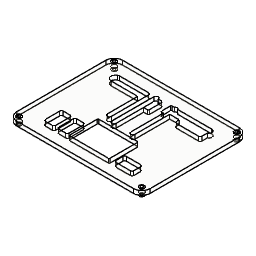
CASE TAMPA (Autodesk Fusion 360 design; units mm, degrees)
Autodesk Fusion 360 part; units mm, degrees
sketch "Esboço1" plane through (0, 0, 0) normal (0, 0, 1) x (1, 0, 0)
  arc A0 through (-111.4942, 26.079, 1.5525) (-112.9084, 25.4932, 1.5525) (-113.4942, 24.079, 1.5525)
  line L0 (-107.2442, 26.079, 1.5525) -> (-102.9942, 26.079, 1.5525)
  line L1 (-126.339, 4.5975, 1.5525) -> (-119.189, 4.5975, 1.5525)
  line L2 (-155, 19.05, 1.5525) -> (-155, -2.46, 1.5525)
  line L3 (-126.339, 4.5975, 1.5525) -> (-127.689, 4.5975, 1.5525)
  line L4 (-117.189, 6.5975, 1.5525) -> (-117.189, 6.7613, 1.5525)
  arc A1 through (-117.189, 24.079, 1.5525) (-117.7748, 25.4932, 1.5525) (-119.189, 26.079, 1.5525)
  arc A2 through (-127.689, 26.079, 1.5525) (-129.1032, 25.4932, 1.5525) (-129.689, 24.079, 1.5525)
  arc A3 through (-119.189, 4.5975, 1.5525) (-117.7748, 5.1833, 1.5525) (-117.189, 6.5975, 1.5525)
  line L5 (-129.689, 24.079, 1.5525) -> (-129.689, 6.5975, 1.5525)
  arc A4 through (-129.689, 6.5975, 1.5525) (-129.1032, 5.1833, 1.5525) (-127.689, 4.5975, 1.5525)
  arc A5 through (-44.2048, 6.3065, 1.5525) (-43.619, 4.8923, 1.5525) (-42.2048, 4.3065, 1.5525)
  line L6 (-42.2048, 4.3065, 1.5525) -> (-24.7233, 4.3065, 1.5525)
  line L7 (-24.7233, 16.8065, 1.5525) -> (-24.8871, 16.8065, 1.5525)
  line L8 (-22.7233, 7.6565, 1.5525) -> (-22.7233, 14.8065, 1.5525)
  arc A6 through (-42.2048, 16.8065, 1.5525) (-43.619, 16.2207, 1.5525) (-44.2048, 14.8065, 1.5525)
  arc A7 through (-22.7233, 14.8065, 1.5525) (-23.3091, 16.2207, 1.5525) (-24.7233, 16.8065, 1.5525)
  line L9 (-22.7233, 7.6565, 1.5525) -> (-22.7233, 6.3065, 1.5525)
  arc A8 through (-24.7233, 4.3065, 1.5525) (-23.3091, 4.8923, 1.5525) (-22.7233, 6.3065, 1.5525)
  line L10 (-44.2048, 6.3065, 1.5525) -> (-44.2048, 14.8065, 1.5525)
  arc A9 through (-17.6621, 90.086, 1.5525) (-15.5638, 94.0019, 1.5525) (-18.997, 96.8215, 1.5525)
  arc A10 through (-68.3, 85.39, 1.5525) (-68.0071, 84.6829, 1.5525) (-67.3, 84.39, 1.5525)
  line L11 (-22.607, 81.481, 1.5525) -> (-24.217, 81.481, 1.5525)
  arc A11 through (-19.6621, 81.481, 1.5525) (-18.2479, 82.0668, 1.5525) (-17.6621, 83.481, 1.5525)
  arc A12 through (-17.6621, 90.086, 1.5525) (-15.5638, 94.0019, 1.5525) (-18.997, 96.8215, 1.5525)
  line L12 (-60.03, 86.9647, 1.5525) -> (-48.617, 86.9647, 1.5525)
  line L13 (-46.617, 81.481, 1.5525) -> (-24.217, 81.481, 1.5525)
  circle A13 through (2.3255, 108.5355, 1.5525) (-2.1745, 111.1336, 1.5525) (-2.1745, 105.9375, 1.5525)
  circle A14 through (0.8255, 108.5355, 1.5525) (-1.4245, 109.8346, 1.5525) (-1.4245, 107.2365, 1.5525)
  arc A15 through (5.79, 105, 1.5525) (2.8611, 112.0711, 1.5525) (-4.21, 115, 1.5525)
  line L14 (-67.3, 84.39, 1.5525) -> (-65.03, 84.39, 1.5525)
  line L15 (-68.3, 94.89, 1.5525) -> (-68.3, 85.39, 1.5525)
  arc A16 through (-60.2097, 96.8205, 1.5525) (-62.3654, 98.3844, 1.5525) (-64.7079, 97.1172, 1.5525)
  line L16 (-48.617, 86.9647, 1.5525) -> (-48.617, 83.481, 1.5525)
  line L17 (-46.617, 81.481, 1.5525) -> (-24.217, 81.481, 1.5525)
  line L18 (-18.997, 96.8215, 1.5525) -> (-60.1253, 96.8215, 1.5525)
  arc A17 through (-48.617, 83.481, 1.5525) (-48.0312, 82.0668, 1.5525) (-46.617, 81.481, 1.5525)
  line L19 (-145, 115, 1.5525) -> (-4.21, 115, 1.5525)
  line L20 (2.8611, 112.0711, 1.5525) -> (7.8611, 112.0711, 1.5525) construction
  arc A18 through (-60.2097, 96.8205, 1.5525) (-62.3654, 98.3844, 1.5525) (-64.7079, 97.1172, 1.5525)
  line L21 (-18.997, 96.8215, 1.5525) -> (-60.1253, 96.8215, 1.5525)
  line L22 (-140, 100, 1.5525) -> (-9.21, 100, 1.5525)
  line L23 (-140, 100, 1.5525) -> (-9.21, 100, 1.5525)
  arc A19 through (-145, 115, 1.5525) (-152.0711, 112.0711, 1.5525) (-155, 105, 1.5525)
  arc A20 through (-48.617, 83.481, 1.5525) (-48.0312, 82.0668, 1.5525) (-46.617, 81.481, 1.5525)
  line L24 (-82.89, 45.09, 1.5525) -> (-82.89, 78.39, 1.5525)
  line L25 (-140, 100, 1.5525) -> (-140, 19.05, 1.5525)
  line L26 (-64.7079, 97.1172, 1.5525) -> (-67.3, 97.1172, 1.5525)
  arc A21 through (-60.1253, 96.8215, 1.5525) (-60.1675, 96.8212, 1.5525) (-60.2097, 96.8205, 1.5525)
  line L27 (-19.6621, 81.481, 1.5525) -> (-22.607, 81.481, 1.5525)
  line L28 (-68.3, 96.1172, 1.5525) -> (-68.3, 94.4279, 1.5525)
  line L29 (-17.6621, 90.086, 1.5525) -> (-17.6621, 83.481, 1.5525)
  circle A22 through (-145.5355, 108.5355, 1.5525) (-150.0355, 111.1336, 1.5525) (-150.0355, 105.9375, 1.5525)
  line L30 (-67.3, 84.39, 1.5525) -> (-65.03, 84.39, 1.5525)
  line L31 (-97.61, 4.09, 1.5525) -> (-51.11, 4.09, 1.5525)
  arc A23 through (-82.89, 95.89, 1.5525) (-85.39, 98.39, 1.5525) (-87.89, 95.89, 1.5525)
  line L32 (-82.89, 95.89, 1.5525) -> (-79.12, 95.89, 1.5525)
  arc A24 through (-77.12, 93.89, 1.5525) (-77.7058, 95.3042, 1.5525) (-79.12, 95.89, 1.5525)
  arc A25 through (-78.12, 78.39, 1.5525) (-77.4129, 78.6829, 1.5525) (-77.12, 79.39, 1.5525)
  line L33 (-78.12, 78.39, 1.5525) -> (-82.89, 78.39, 1.5525)
  line L34 (-82.89, 95.89, 1.5525) -> (-79.12, 95.89, 1.5525)
  line L35 (-100.507, 96.7775, 1.5525) -> (-130.197, 96.7775, 1.5525)
  line L36 (-87.89, 95.89, 1.5525) -> (-87.89, 45.09, 1.5525)
  line L37 (-140, 2.54, 1.5525) -> (-9.21, 2.54, 1.5525)
  arc A26 through (-132.0334, 96.2971, 1.5525) (-135.2196, 90.596, 1.5525) (-130.197, 86.4212, 1.5525)
  line L38 (-48.617, 86.9647, 1.5525) -> (-48.617, 83.481, 1.5525)
  arc A27 through (-68.3, 85.39, 1.5525) (-68.0071, 84.6829, 1.5525) (-67.3, 84.39, 1.5525)
  line L39 (-100.507, 96.7775, 1.5525) -> (-95.03, 96.7775, 1.5525)
  arc A28 through (-78.12, 78.39, 1.5525) (-77.4129, 78.6829, 1.5525) (-77.12, 79.39, 1.5525)
  line L40 (-140, 100, 1.5525) -> (-130.197, 100, 1.5525)
  line L41 (-68.3, 94.89, 1.5525) -> (-68.3, 85.39, 1.5525)
  arc A29 through (-93.03, 94.7775, 1.5525) (-93.6158, 96.1917, 1.5525) (-95.03, 96.7775, 1.5525)
  line L42 (-140, 100, 1.5525) -> (-130.197, 100, 1.5525)
  line L43 (-97.61, 39.09, 1.5525) -> (-51.11, 39.09, 1.5525)
  line L44 (-152.0711, 112.0711, 1.5525) -> (-147.0711, 112.0711, 1.5525) construction
  line L45 (-130.197, 86.4212, 1.5525) -> (-98.03, 86.4212, 1.5525)
  line L46 (-100.507, 96.7775, 1.5525) -> (-95.03, 96.7775, 1.5525)
  line L47 (-77.12, 93.89, 1.5525) -> (-77.12, 79.39, 1.5525)
  arc A30 through (-60.1253, 96.8215, 1.5525) (-60.1675, 96.8212, 1.5525) (-60.2097, 96.8205, 1.5525)
  arc A31 through (-67.3, 97.1172, 1.5525) (-68.0071, 96.8244, 1.5525) (-68.3, 96.1172, 1.5525)
  line L48 (-77.12, 93.89, 1.5525) -> (-77.12, 79.39, 1.5525)
  line L49 (-78.12, 78.39, 1.5525) -> (-82.89, 78.39, 1.5525)
  arc A32 through (-82.89, 95.89, 1.5525) (-85.39, 98.39, 1.5525) (-87.89, 95.89, 1.5525)
  arc A33 through (-77.12, 93.89, 1.5525) (-77.7058, 95.3042, 1.5525) (-79.12, 95.89, 1.5525)
  arc A34 through (-130.197, 96.7775, 1.5525) (-131.1461, 96.6554, 1.5525) (-132.0334, 96.2971, 1.5525)
  arc A35 through (-93.03, 94.7775, 1.5525) (-93.6158, 96.1917, 1.5525) (-95.03, 96.7775, 1.5525)
  circle A36 through (-147.0355, 108.5355, 1.5525) (-149.2855, 109.8346, 1.5525) (-149.2855, 107.2365, 1.5525)
  line L50 (2.8611, -9.5311, 1.5525) -> (7.8611, -9.5311, 1.5525) construction
  line L51 (-50.11, 5.09, 1.5525) -> (-50.11, 38.09, 1.5525)
  arc A37 through (-65.03, 45.09, 1.5525) (-62.53, 42.59, 1.5525) (-60.03, 45.09, 1.5525)
  circle A38 through (2.3255, -5.9955, 1.5525) (-2.1745, -3.3975, 1.5525) (-2.1745, -8.5936, 1.5525)
  line L52 (5.79, -2.46, 1.5525) -> (5.79, 19.05, 1.5525)
  line L53 (-145, -12.46, 1.5525) -> (-4.21, -12.46, 1.5525)
  line L54 (-9.21, 2.54, 1.5525) -> (-9.21, 19.05, 1.5525)
  arc A39 through (-50.11, 38.09, 1.5525) (-50.4029, 38.7971, 1.5525) (-51.11, 39.09, 1.5525)
  circle A40 through (0.8255, -5.9955, 1.5525) (-1.4245, -4.6965, 1.5525) (-1.4245, -7.2946, 1.5525)
  arc A41 through (-65.03, 45.09, 1.5525) (-62.53, 42.59, 1.5525) (-60.03, 45.09, 1.5525)
  arc A42 through (-4.21, -12.46, 1.5525) (2.8611, -9.5311, 1.5525) (5.79, -2.46, 1.5525)
  arc A43 through (-51.11, 4.09, 1.5525) (-50.4029, 4.3829, 1.5525) (-50.11, 5.09, 1.5525)
  line L55 (-24.7233, 16.8065, 1.5525) -> (-42.2048, 16.8065, 1.5525)
  arc A44 through (-102.9942, 4.5975, 1.5525) (-101.58, 5.1833, 1.5525) (-100.9942, 6.5975, 1.5525)
  line L56 (-117.189, 6.5975, 1.5525) -> (-117.189, 24.079, 1.5525)
  line L57 (-111.4942, 4.5975, 1.5525) -> (-102.9942, 4.5975, 1.5525)
  line L58 (-127.689, 26.079, 1.5525) -> (-119.189, 26.079, 1.5525)
  line L59 (-113.4942, 24.079, 1.5525) -> (-113.4942, 6.5975, 1.5525)
  line L60 (-140, 2.54, 1.5525) -> (-126.339, 2.54, 1.5525)
  arc A45 through (-97.61, 39.09, 1.5525) (-98.3171, 38.7971, 1.5525) (-98.61, 38.09, 1.5525)
  line L61 (-98.61, 5.09, 1.5525) -> (-98.61, 38.09, 1.5525)
  line L62 (-152.0711, -9.5311, 1.5525) -> (-147.0711, -9.5311, 1.5525) construction
  arc A46 through (-87.89, 45.09, 1.5525) (-85.39, 42.59, 1.5525) (-82.89, 45.09, 1.5525)
  circle A47 through (-147.0355, -5.9955, 1.5525) (-149.2855, -4.6965, 1.5525) (-149.2855, -7.2946, 1.5525)
  arc A48 through (-98.03, 49.53, 1.5525) (-95.53, 47.03, 1.5525) (-93.03, 49.53, 1.5525)
  line L63 (-140, 19.05, 1.5525) -> (-140, 2.54, 1.5525)
  arc A49 through (-87.89, 45.09, 1.5525) (-85.39, 42.59, 1.5525) (-82.89, 45.09, 1.5525)
  arc A50 through (-98.03, 49.53, 1.5525) (-95.53, 47.03, 1.5525) (-93.03, 49.53, 1.5525)
  arc A51 through (-98.61, 5.09, 1.5525) (-98.3171, 4.3829, 1.5525) (-97.61, 4.09, 1.5525)
  circle A52 through (-145.5355, -5.9955, 1.5525) (-150.0355, -3.3975, 1.5525) (-150.0355, -8.5936, 1.5525)
  line L64 (-140, 2.54, 1.5525) -> (-98.61, 2.54, 1.5525)
  arc A53 through (-155, -2.46, 1.5525) (-152.0711, -9.5311, 1.5525) (-145, -12.46, 1.5525)
  line L65 (-9.21, 100, 1.5525) -> (-9.21, 19.05, 1.5525)
  line L66 (-82.89, 45.09, 1.5525) -> (-82.89, 78.39, 1.5525)
  line L67 (-60.03, 45.09, 1.5525) -> (-60.03, 86.9647, 1.5525)
  line L68 (-9.21, 100, 1.5525) -> (-9.21, 19.05, 1.5525)
  line L69 (-140, 100, 1.5525) -> (-140, 19.05, 1.5525)
  line L70 (-65.03, 84.39, 1.5525) -> (-65.03, 45.09, 1.5525)
  line L71 (-140, 100, 1.5525) -> (-140, 19.05, 1.5525)
  line L72 (-87.89, 95.89, 1.5525) -> (-87.89, 45.09, 1.5525)
  line L73 (-65.03, 84.39, 1.5525) -> (-65.03, 45.09, 1.5525)
  line L74 (-140, 100, 1.5525) -> (-140, 19.05, 1.5525)
  line L75 (-60.03, 45.09, 1.5525) -> (-60.03, 86.9647, 1.5525)
  line L76 (-93.03, 49.53, 1.5525) -> (-93.03, 94.7775, 1.5525)
  line L77 (-98.03, 86.4212, 1.5525) -> (-98.03, 49.53, 1.5525)
  line L78 (-98.03, 86.4212, 1.5525) -> (-98.03, 49.53, 1.5525)
  line L79 (-9.21, 100, 1.5525) -> (-9.21, 19.05, 1.5525)
  line L80 (5.79, 105, 1.5525) -> (5.79, 19.05, 1.5525)
  line L81 (-93.03, 49.53, 1.5525) -> (-93.03, 94.7775, 1.5525)
  line L82 (-9.21, 100, 1.5525) -> (-9.21, 19.05, 1.5525)
  line L83 (-155, 105, 1.5525) -> (-155, 19.05, 1.5525)
  arc A54 through (-113.4942, 6.5975, 1.5525) (-112.9084, 5.1833, 1.5525) (-111.4942, 4.5975, 1.5525)
  line L84 (-100.9942, 24.079, 1.5525) -> (-100.9942, 6.5975, 1.5525)
  line L85 (-107.2442, 26.079, 1.5525) -> (-111.4942, 26.079, 1.5525)
  arc A55 through (-100.9942, 24.079, 1.5525) (-101.58, 25.4932, 1.5525) (-102.9942, 26.079, 1.5525)
  point P0 (-68.3, 95.89)
  point P1 (-22.217, 81.481)
  point P2 (-77.12, 78.39)
  point P3 (-100.9942, 26.079)
  point P4 (-50.11, 39.09)
  point P5 (-50.11, 4.09)
  point P6 (-68.3, 84.39)
  point P7 (-140, 0)
  point P8 (-98.61, 4.09)
  point P9 (-48.617, 81.481)
  point P10 (-77.12, 95.89)
  point P11 (-38.3259, -0.1301)
  point P12 (-68.3, 95.89)
  point P13 (-77.12, 95.89)
  point P14 (-77.12, 78.39)
  point P15 (-68.3, 84.39)
  point P16 (-48.617, 81.481)
  point P17 (-22.217, 81.481)
  point P18 (-113.4942, 26.079)
  dimension "d389" = 130.79
  dimension "d390" = 80.95
  dimension "d391" = 130.79
  dimension "d392" = 80.95
  dimension "d393" = 9.803
  dimension "d394" = 7.5
  dimension "d395" = 5
  dimension "d396" = 5
  dimension "d397" = 5
  dimension "d398" = 17.5
  dimension "d399" = 1
  dimension "d400" = 2
  dimension "d401" = 11.5
  dimension "d402" = 7
  dimension "d403" = 26.4
  dimension "d404" = 2
  dimension "d405" = 2
  dimension "d406" = 130.79
  dimension "d407" = 130.79
  dimension "d408" = 9.803
  dimension "d409" = 5
  dimension "d410" = 5
  dimension "d411" = 5
  dimension "d412" = 17.5
  dimension "d413" = 1
  dimension "d414" = 2
  dimension "d415" = 11.5
  dimension "d416" = 7
  dimension "d417" = 26.4
  dimension "d418" = 2
  dimension "d419" = 2
  dimension "d420" = 16.51
  dimension "d421" = 15
  dimension "d422" = 15
  dimension "d423" = 15
  dimension "d424" = 15
  dimension "d425" = 15
  dimension "d426" = 15
  dimension "d427" = 10
  dimension "d428" = 5
  dimension "d429" = 5
  dimension "d430" = 5
  dimension "d431" = 5
  dimension "d432" = 3
  dimension "d433" = 6
  dimension "d434" = 3
  dimension "d435" = 6
  dimension "d436" = 3
  dimension "d437" = 6
  dimension "d438" = 3
  dimension "d439" = 6
  dimension "d440" = 1
  dimension "d441" = 2
  dimension "d442" = 1.55
  dimension "d443" = 48.5
  dimension "d444" = 35
  dimension "d445" = 1
  dimension "d446" = 1
  dimension "d447" = 6.25
  dimension "d448" = 6.25
  dimension "d449" = 2
  dimension "d450" = 2
  measures "d398" distance of P13 P14
  measures "d401" distance of P12 P15
  measures "d403" distance of P16 P17
  measures "d412" distance of P14 P13
  measures "d415" distance of P12 P15
  measures "d417" distance of P17 P16
  measures "d443" distance of P5 P8
  measures "d444" distance of P4 P5
extrude "Extrusão2" add sketch "Esboço1" against normal blind 3 contours A13 | A22 | A38 | A52 in plane through (0, 0, 1.5525) normal (0, 0, 1) makes body 1 at (-150.5206, 106.2862, -0.4475) makes body 2 at (2.3218, -6.1451, -0.4475) makes body 3 at (-145.5393, -6.1451, -0.4475) makes body 4 at (2.1446, 107.5095, -0.4475)
extrude "Extrusão3" add sketch "Esboço1" along normal blind 5 separate body contours L2 A15 L19 A19 L52 L53 A42 A53 L80 L83 | L22 L23 L25 L37 L40 L42 L54 L60 L63 L64 L65 L68 L69 L71 L74 L79 L82 in plane through (0, 0, 1.5525) normal (0, 0, 1) makes body 5
extrude "Extrusão4" add sketch "Esboço1" along normal blind 5.5 contours A13 | A22 | A38 | A52 in plane through (0, 0, 1.5525) normal (0, 0, 1) bodies 1 2 3 4 5
extrude "Extrusão1" [suppressed]
sketch "Esboço2" plane through (0, 0, 0) normal (0, 0, 1) x (1, 0, 0)
  line L0 (-73.4978, 88.47) -> (-73.4978, 35)
  arc A0 (-73.4978, 35) -> (-68.4978, 35) centre (-70.9978, 35) ccw
  line L1 (-68.4978, 35) -> (-68.4978, 88.47)
  arc A1 (-68.4978, 88.47) -> (-73.4978, 88.47) centre (-70.9978, 88.47) ccw
  line L2 (-64.8478, 88.47) -> (-64.8478, 35)
  arc A2 (-64.8478, 35) -> (-59.8478, 35) centre (-62.3478, 35) ccw
  line L3 (-59.8478, 35) -> (-59.8478, 88.47)
  arc A3 (-59.8478, 88.47) -> (-64.8478, 88.47) centre (-62.3478, 88.47) ccw
  constraint tangent L0 A0
  constraint tangent A0 L1
  constraint parallel L0 L1
  constraint tangent L1 A1
  constraint tangent L0 A1
  constraint tangent L2 A2
  constraint tangent A2 L3
  constraint parallel L2 L3
  constraint tangent L3 A3
  constraint tangent L2 A3
